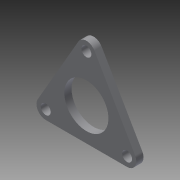
# Autodesk Inventor part: BackupPlate
Saved by Autodesk Inventor 2014 SP1 (Build 180222100, 222)
## iProperties
Created: 2013-12-26
Part Number: BackupPlate
Material: Generic
Document SubType Name: Modeling
Designer: Jack
Density: 1 g/cm^3
Appearance: Default
Author: Jack
Autodesk Inventor part; units mm, degrees
ref_plane "YZ Plane" through (0, 0, 0) normal (1, 0, 0) x (0, 1, 0)
ref_plane "XZ Plane" through (0, 0, 0) normal (0, 1, 0) x (-1, 0, 0)
ref_plane "XY Plane" through (0, 0, 0) normal (0, 0, 1) x (1, 0, 0)
sketch "Sketch1" plane through (0, 0, 0) normal (0, 1, 0) x (-1, 0, 0)
  circle A0 centre (0, 0) radius 16.5 construction
  circle A1 centre (0, 0) radius 7.75
  line L0 (0, 0) -> (14.2894, -8.25) construction
  line L1 (0, 0) -> (-14.2894, -8.25) construction
  line L2 (-16.5, 0) -> (16.5, 0) construction
  circle A2 centre (14.2894, -8.25) radius 1.75
  circle A3 centre (-14.2894, -8.25) radius 1.75
  circle A4 centre (0, 16.5) radius 1.75
  circle A5 centre (-14.2894, -8.25) radius 3.25 construction
  circle A6 centre (14.2894, -8.25) radius 3.25 construction
  circle A7 centre (0, 16.5) radius 3.25 construction
  line L3 (14.2894, -11.5) -> (-14.2894, -11.5)
  line L4 (17.104, -6.625) -> (2.8146, 18.125)
  line L5 (-17.104, -6.625) -> (-2.8146, 18.125)
  arc A8 (-17.104, -6.625) -> (-14.2894, -11.5) centre (-14.2894, -8.25) ccw
  arc A9 (14.2894, -11.5) -> (17.104, -6.625) centre (14.2894, -8.25) ccw
  arc A10 (2.8146, 18.125) -> (-2.8146, 18.125) centre (0, 16.5) ccw
  dimension "d0" = 33
  dimension "d1" = 15.5
  dimension "d2" = 30
  dimension "d3" = 30
  dimension "d4" = 3.5
  dimension "d5" = 3.5
  dimension "d6" = 3.5
  dimension "d7" = 6.5
  dimension "d8" = 6.5
  dimension "d9" = 6.5
  constraints: 17 point on circle, 12 end point, 11 centre point, 10 coincident, 6 tangent, 1 horizontal, 1 midpoint, 1 vertical alignment
  measures "d0" diameter of A0
  measures "d1" diameter of A1
  measures "d2" angle of L1 L2
  measures "d3" angle of L2 L0
  measures "d4" diameter of A2
  measures "d5" diameter of A3
  measures "d6" diameter of A4
  measures "d7" diameter of A5
  measures "d8" diameter of A6
  measures "d9" diameter of A7
extrude "Extrusion1" add sketch "Sketch1" along normal blind 2.54
body "Solid1"
